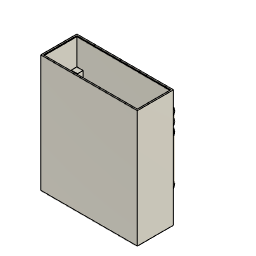
Electronics box (Autodesk Fusion 360 design; units mm, degrees)
Autodesk Fusion 360 part; units mm, degrees
sketch "Sketch1" plane through (0, 0, 0) normal (0, 0, 1) x (1, 0, 0)
  line L0 (0, 0) -> (107, 0)
  line L1 (107, 0) -> (107, 40)
  line L2 (107, 40) -> (0, 40)
  line L3 (0, 40) -> (0, 0)
  line L4 (2, 38) -> (105, 38)
  line L5 (105, 38) -> (105, 2)
  line L6 (105, 2) -> (2, 2)
  line L7 (105, 20) -> (107, 20) construction
  line L8 (0, 20) -> (2, 20) construction
  line L9 (53.5, 38) -> (53.5, 40) construction
  line L10 (53.5, 2) -> (53.5, 0) construction
  line L11 (2, 31) -> (9, 31)
  line L12 (9, 31) -> (9, 29)
  line L13 (9, 29) -> (2, 29)
  line L14 (2, 29) -> (2, 31)
  line L15 (2, 30.99) -> (2, 38)
  line L16 (2, 29.0121) -> (2, 30.99)
  line L17 (53.5, 38) -> (53.5, 2) construction
  line L18 (53.5, 40) -> (53.5, 80.2877) construction
  circle A0 centre (53.5, 65.9111) radius 20.5
  circle A1 centre (53.5, 65.9111) radius 12.5
  line L19 (53.5, 65.9111) -> (74, 65.9111) construction
  line L20 (53.5, 65.9111) -> (33, 65.9111) construction
  arc A2 (0, 40) -> (33, 65.9111) centre (0, 73.9697) ccw
  arc A3 (74, 65.9111) -> (107, 40) centre (107, 73.9697) ccw
  line L21 (54.5, 78.371) -> (54.5, 86.3867)
  line L22 (52.5, 78.371) -> (52.5, 86.3867)
  line L23 (53.5, 75.2968) -> (54.5, 75.2968) construction
  line L24 (53.5, 75.2968) -> (52.5, 75.2968) construction
  circle A4 centre (53.5, 65.9111) radius 19
  line L25 (9, 31) -> (9, 38)
  line L26 (9, 2) -> (9, 4)
  line L27 (9, 4) -> (9, 29)
  line L28 (2, 2) -> (2, 29)
  line L29 (98, 38) -> (98, 2)
  line L30 (2, 20) -> (105, 20) construction
  line L31 (98, 4) -> (105, 4)
  line L32 (2, 4) -> (9, 4)
  line L33 (5.5, 4) -> (5.5, 29) construction
  circle A5 centre (5.5, 20) radius 2.1
  line L34 (105, 31) -> (98, 31)
  line L35 (105, 29) -> (98, 29)
  line L36 (101.5, 29) -> (101.5, 4) construction
  circle A6 centre (101.5, 20) radius 2.1
  dimension "d1" = 107
  dimension "d2" = 40
  dimension "d7" = 2
  dimension "d10" = 2
  dimension "d15" = 2
  dimension "d53" = 41
  dimension "d54" = 25
  dimension "d56" = 2
  dimension "d61" = 38
  dimension "d73" = 7
  dimension "d75" = 7
  dimension "d76" = 7
  dimension "d83" = 2
  dimension "d84" = 2
  dimension "d85" = 4.2
  dimension "d87" = 25
  dimension "d88" = 2
  dimension "d89" = 7
  dimension "d90" = 4.2
  constraint horizontal L0
  constraint vertical L1
  constraint horizontal L2
  constraint vertical L3
  constraint coincident L0.start L3.end
  constraint horizontal L4
  constraint vertical L5
  constraint horizontal L6
  constraint midpoint L5 L7.start
  constraint coincident L1 L7.end
  constraint perpendicular L1 L7
  constraint midpoint L3 L8.start
  constraint equal L7 L8
  constraint midpoint L4 L9.start
  constraint midpoint L2 L9.end
  constraint midpoint L6 L10.start
  constraint midpoint L0 L10.end
  constraint equal L9 L10
  constraint horizontal L11
  constraint vertical L12
  constraint horizontal L13
  constraint vertical L14
  constraint perpendicular L2 L18
  constraint coincident L18 A0.centre
  constraint concentric A0 A1
  constraint coincident A0.centre A1.centre
  constraint coincident A0 L19.end
  constraint perpendicular L18 L19
  constraint coincident A0 L20.end
  constraint perpendicular L18 L20
  constraint tangent L2 A2
  constraint tangent L2 A3
  constraint coincident A1 L21.start
  constraint coincident A0 L21.end
  constraint parallel L18 L21
  constraint coincident A0 L22.end
  constraint parallel L18 L22
  constraint coincident L18 L23.start
  constraint coincident L21 L23.end
  constraint perpendicular L21 L23
  constraint coincident L22 L24.end
  constraint perpendicular L22 L24
  constraint equal L23 L24
  constraint coincident A1 L22.start
  constraint concentric A1 A4
  constraint coincident L4 L25.end
  constraint perpendicular L4 L25
  constraint coincident L6 L26.start
  constraint perpendicular L6 L26
  constraint perpendicular L13 L27
  constraint perpendicular L8 L28
  constraint coincident L4 L29.start
  constraint coincident L6 L29.end
  constraint perpendicular L6 L29
  constraint perpendicular L5 L30
  constraint coincident L29 L31.start
  constraint coincident L5 L31.end
  constraint perpendicular L5 L31
  constraint coincident L28 L32.start
  constraint coincident L27 L26.end
  constraint perpendicular L27 L32
  constraint midpoint L32 L33.start
  constraint midpoint L13 L33.end
  constraint coincident L30 A5.centre
  constraint coincident L33 A5.centre
  constraint coincident L5 L34.start
  constraint coincident L29 L34.end
  constraint perpendicular L29 L34
  constraint coincident L5 L35.start
  constraint coincident L29 L35.end
  constraint perpendicular L29 L35
  constraint midpoint L35 L36.start
  constraint midpoint L31 L36.end
  constraint coincident L36 A6.centre
  constraint coincident L30 A6.centre
  measures "d1" distance of L0.start L0.end
  measures "d2" distance of L0.start L2.end
  measures "d7" distance of L9.start L9.end
  measures "d10" distance of L11 L13
  measures "d15" distance of L3 L15
  measures "d53" diameter of A0
  measures "d54" diameter of A1
  measures "d56" distance of L21 L22
  measures "d61" diameter of A4
  measures "d73" distance of L4 L11
  measures "d75" distance of L11.start L11.end
  measures "d76" distance of L5 L29
  measures "d83" distance of L6 L31
  measures "d84" distance of L6 L32
  measures "d85" diameter of A5
  measures "d87" distance of L13 L32
  measures "d88" distance of L34 L35
  measures "d89" distance of L4 L34
  measures "d90" diameter of A6
extrude "Extrude1" add sketch "Sketch1" along normal blind 130 contours L0 L1 L2 L3 | L4 L11 L15 L25 | L4 L6 L12 L25 L26 L27 L29 | L11 L12 L13 L14 L15 L16 | L4 L5 L29 L34 | L5 L29 L34 L35 | L13 L27 L28 L32 | L5 L29 L31 L35 | L6 L26 L28 L32 | L5 L6 L29 L31 | A5 | A6
shell "Shell1" thickness 2 removed faces 1 at (71.3333, 26.6667, 130)
extrude "Extrude5" add sketch "Sketch1" along normal blind 50 contours L2 A0 A2 A3 | A0 L21 L22 A4 | A1 L21 L22 A4 picked at (35.9552, 57.4776) picked at (37.4613, 60.9117)
fillet "Fillet1" radius 10 1 edges at (53.5, 40, 50)
extrude "Extrude6" cut sketch "Sketch1" along normal blind 6 from surface at 50 contours A1 L21 L22 A4 picked at (37.4613, 60.9117)
extrude "Extrude7" add sketch "Sketch1" along normal blind 10 from surface at 50 contours A1 L21 L22 A4 picked at (37.4613, 60.9117)
extrude "Extrude8" add sketch "Sketch1" along normal blind 10 from surface at 60 contours A0 L21 L22 A4 | A1 L21 L22 A4 picked at (35.9552, 57.4776) picked at (37.4613, 60.9117)
fillet "Fillet2" radius 1 4 edges at (71.8477, 70.8469, 50) (53.5, 46.9111, 50.489) (35.1523, 70.8469, 50) (53.5, 46.9111, 60)
extrude "Extrude9" add sketch "Sketch1" along normal blind 100.5 contours L4 L11 L15 L25 | L4 L5 L29 L34 | L13 L27 L28 L32 | L5 L29 L31 L35 | A5 | A6
extrude "Extrude10" cut sketch "Sketch1" against normal blind 10 from surface at 100.5 contours A5 | A6
chamfer "Chamfer1" distance 0.3 angle 45 1 edges at (3.5421, 20.7594, 100.5)
chamfer "Chamfer2" distance 0.7 distance2 1.3 6 edges at (101.5, 4, 100.5) (101.5, 29, 100.5) (101.5, 31, 100.5) (5.5, 4, 100.5) (5.5, 29, 100.5) (5.5, 31, 100.5) measured on face at (101.4477, 8.6353, 100.5) measured on face at (101.4477, 8.6353, 100.5) measured on face at (100.3333, 35.6667, 100.5) measured on face at (5.4402, 8.5356, 100.5) measured on face at (5.4402, 8.5356, 100.5) measured on face at (4.3333, 35.6667, 100.5)
chamfer "Chamfer3" distance 0.5 angle 45 4 edges at (53.5, 38, 130) (2, 20, 130) (53.5, 2, 130) (105, 20, 130)
chamfer "Chamfer4" distance 0.5 angle 45 1 edges at (53.5, 53.4111, 70)
chamfer "Chamfer5" distance 0.5 angle 45 1 edges at (53.5, 53.4111, 0)
